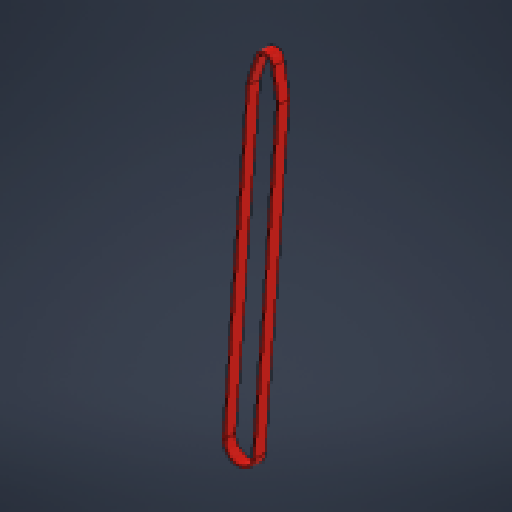
# Autodesk Inventor part: Triple Indexer band
Saved by Autodesk Inventor 2023.2 (Build 272271030, 271C)
## iProperties
Created: 2023-04-07
Part Number: Triple Indexer band
Material: Generic
Document SubType Name: Modeling
Designer: Main Account
Density: 1 g/cm^3
Appearance: Default
Author: Main Account
Autodesk Inventor part; units mm, degrees
ref_plane "YZ Plane" through (0, 0, 0) normal (1, 0, 0) x (0, 1, 0)
ref_plane "XZ Plane" through (0, 0, 0) normal (0, 1, 0) x (-1, 0, 0)
ref_plane "XY Plane" through (0, 0, 0) normal (0, 0, 1) x (1, 0, 0)
sketch "Sketch1" plane through (0, 0, 0) normal (0, 0, 1) x (1, 0, 0)
  circle A0 centre (6, 6) radius 6.35 construction
  arc A1 (-0.3319, 6.4786) -> (12.3319, 5.5214) centre (6, 6) ccw
  circle A2 centre (18.014, 164.9586) radius 6.35 construction
  arc A3 (21.1506, 165.4511) -> (14.9871, 165.917) centre (18.014, 164.9586) ccw
  line L0 (10.6933, 152.3554) -> (10.6053, 151.1903) construction
  line L1 (23.3572, 151.3983) -> (23.2692, 150.2332) construction
  line L2 (23.3572, 151.3983) -> (21.1506, 165.4511)
  line L3 (14.9871, 165.917) -> (10.6933, 152.3554)
  line L4 (23.3572, 151.3983) -> (23.2692, 150.2332)
  line L5 (10.6933, 152.3554) -> (10.6053, 151.1903)
  line L6 (10.6053, 151.1903) -> (-0.3319, 6.4786)
  line L7 (12.3319, 5.5214) -> (23.2692, 150.2332)
  line L8 (13.35, 129.2896) -> (13.35, 130.5741)
  line L9 (-1.35, 130.5741) -> (-1.35, 129.2896)
  line L10 (24.2663, 150.1578) -> (24.3631, 151.4387)
  line L11 (24.3631, 151.4387) -> (22.1385, 165.6063)
  arc A4 (22.1385, 165.6063) -> (14.0338, 166.2188) centre (18.014, 164.9586) ccw
  line L12 (14.0338, 166.2188) -> (9.7049, 152.5465)
  line L13 (9.7049, 152.5465) -> (9.6081, 151.2657)
  line L14 (9.6081, 151.2657) -> (-1.3291, 6.5539)
  arc A5 (-1.3291, 6.5539) -> (13.3291, 5.4461) centre (6, 6) ccw
  line L15 (13.3291, 5.4461) -> (24.2663, 150.1578)
  point P0 (0, 0)
  point P1 (8.7925, 140.4734)
  point P2 (9.2272, 146.2258)
  point P3 (8.0394, 130.5099)
  point P4 (9.9436, 147.8903)
  point P5 (10.3642, 148.0002)
  point P6 (9.4208, 148.7872)
  dimension "d0" = 6.35
  dimension "d5" = 1
  constraints: 28 end point, 8 point on circle, 4 centre point, 4 tangent, 2 coincident, 2 collinear, 1 concentric, 7 other
  measures "d0" diameter of A3
  measures "d5" distance between parallel lines of L7 L15
extrude "Extrusion1" add sketch "Sketch1" along normal blind 5
body "Solid1"
